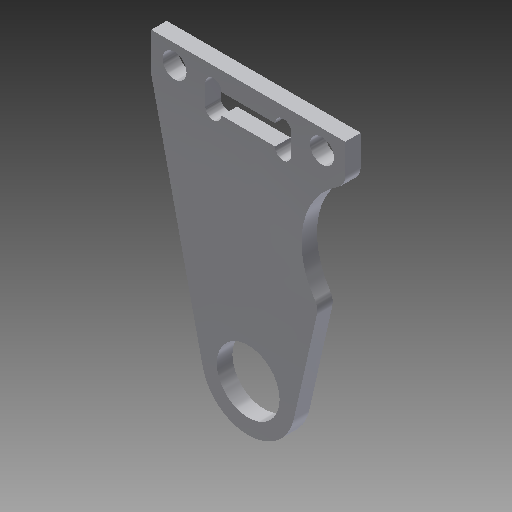
# Autodesk Inventor part: 付け根ロール_サブフレーム_1_2
Saved by Autodesk Inventor 2018 (Build 220112000, 112)
## iProperties
Created: 2016-05-01
Part Number: 付け根ロール_サブフレーム_1_2
Material: アルミニウム 2014-T4
Document SubType Name: Modeling
Designer: hiroaki
Density: 2.8 g/cm^3
Appearance: サテン
Mass: 3.13765 g
Surface Area: 15.014 cm^2
Volume: 1.12059 cm^3
d0: 1.000 ul
d1: 8.100 mm
d2: 6.000 mm
d3: 2.000 mm
d4: 0.00 deg
d5: 25.000 mm
d6: 0.000 mm
Author: hiroaki
Autodesk Inventor part; units mm, degrees
ref_plane "YZ Plane" through (0, 0, 0) normal (1, 0, 0) x (0, 1, 0)
ref_plane "XZ Plane" through (0, 0, 0) normal (0, 1, 0) x (-1, 0, 0)
ref_plane "XY Plane" through (0, 0, 0) normal (0, 0, 1) x (1, 0, 0)
derived "付け根ロール_基礎_2.ipt"
sketch "スケッチ1" plane through (0, 0, 0) normal (0, 0, 1) x (1, 0, 0)
  circle A0 centre (0, 0) radius 5.05 construction
  circle A1 centre (0, 8.5) radius 1.35 construction
  circle A2 centre (-8.5, 0) radius 1.35 construction
  circle A3 centre (0, -8.5) radius 1.35 construction
  circle A4 centre (8.5, 0) radius 1.35 construction
  line L0 (-12.5, 28) -> (-10.9846, -0.5824) construction
  line L1 (-12.5, 28) -> (-12.5, 30.5)
  line L2 (12.5, 28) -> (10.9846, -0.5824) construction
  arc A5 (-10.9846, -0.5824) -> (10.9846, -0.5824) centre (0, 0) ccw construction
  line L3 (12.5, 30.5) -> (-12.5, 30.5) construction
  line L4 (-12.5, 30.5) -> (-12.5, 28) construction
  line L5 (-12.5, 28) -> (12.5, 28) construction
  line L6 (-29.05, 12) -> (29.25, 12) construction
  line L7 (29.25, 12) -> (29.25, -11) construction
  line L8 (29.25, -11) -> (-29.05, -11) construction
  line L9 (-29.05, -11) -> (-29.05, 12) construction
  circle A6 centre (0, 0) radius 31.6159 construction
  circle A7 centre (-9.5, 30.5) radius 1.55
  line L10 (-12.5, 30.5) -> (-12.5, 33)
  line L11 (-12.5, 33) -> (12.5, 33)
  line L12 (12.5, 33) -> (12.5, 30.5)
  line L13 (12.5, 30.5) -> (12.5, 28) construction
  line L14 (12.5, 30.5) -> (12.5, 28)
  line L15 (-5.5, 30.5) -> (5.5, 30.5) construction
  line L16 (5.5, 30.5) -> (5.5, 28) construction
  line L17 (5.5, 28) -> (-5.5, 28) construction
  line L18 (-5.5, 28) -> (-5.5, 30.5) construction
  circle A8 centre (9.5, 30.5) radius 1.55
  line L19 (0, 0) -> (0, 5.5002) construction
  line L20 (5.55, 27.95) -> (5.55, 30.55) construction
  line L21 (5.55, 30.55) -> (-5.55, 30.55) construction
  line L22 (-5.55, 30.55) -> (-5.55, 27.95) construction
  line L23 (-5.55, 27.95) -> (5.55, 27.95) construction
  circle A9 centre (-4.5, 30.55) radius 1.05 construction
  line L24 (-5.55, 30.55) -> (-5.55, 27.95)
  arc A10 (-3.45, 30.55) -> (-5.55, 30.55) centre (-4.5, 30.55) ccw
  line L25 (-3.45, 30.55) -> (3.45, 30.55)
  arc A11 (-5.55, 27.95) -> (-3.45, 27.95) centre (-4.5, 27.95) ccw
  line L26 (5.55, 29.25) -> (-5.55, 29.25) construction
  line L27 (-3.45, 27.95) -> (3.45, 27.95)
  line L28 (5.55, 30.55) -> (5.55, 27.95)
  arc A12 (5.55, 30.55) -> (3.45, 30.55) centre (4.5, 30.55) ccw
  arc A13 (3.45, 27.95) -> (5.55, 27.95) centre (4.5, 27.95) ccw
  circle A14 centre (0, 0) radius 4.05
  line L29 (-12.5, 28) -> (-5.8515, -1.3266)
  line L30 (12.5, 28) -> (5.8515, -1.3266)
  arc A15 (-5.8515, -1.3266) -> (5.8515, -1.3266) centre (0, 0) ccw
  line L31 (-5.55, 30.55) -> (-4.5, 30.55) construction
  circle A16 centre (-9.5, 30.5) radius 3 construction
  point P0 (0, 30.5)
  point P1 (-12.5, 29.25)
  point P2 (0, 30.5)
  point P3 (0, 30.5)
  point P4 (0, 33)
  dimension "d1" = 8.1
  dimension "d2" = 6
  dimension "d5" = 25
  dimension "d6" = 0
  measures "d1" diameter of A14
  measures "d2" radius of A15
  measures "d5" distance of L10.end L11.end
  measures "d6" horizontal distance of L10.end L10.start
extrude "押し出し1" add sketch "スケッチ1" along normal blind 2
sketch "スケッチ3" plane through (-12.5, 33, 2) normal (0, 0, 1) x (1, 0, 0)
  circle A0 centre (12.5, -33) radius 4.05 projected
  line L0 (18.3515, -34.3266) -> (25, -5) projected
  arc A1 (25, -5) -> (21.5449, -20.2403) centre (29.3589, -14) ccw
  dimension "d7" = 10
  dimension "d8" = 19
  constraints: 2 point on circle, 1 centre point, 1 point on line
  measures "d7" radius of A1
  measures "d8" vertical distance of A1.centre A0.centre
extrude "押し出し2" cut sketch "スケッチ3" against normal blind 10 contours A1 L0
fillet "フィレット1" radius 2 2 edges at (9.0449, 12.7597, 1) (12.5, 28, 1)
